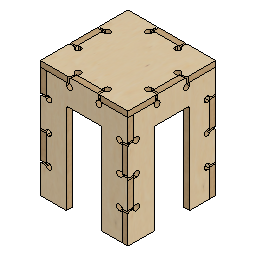
puzzleParam (Autodesk Fusion 360 design; units mm, degrees)
Autodesk Fusion 360 part; units mm, degrees
note: some values were not read from the file. Set by a fixed rule: which sketch regions a step uses.
sketch "Sketch1" plane through (0, 0, 0) normal (0, 0, 1) x (1, 0, 0)
  line L0 (-168.75, 168.75) -> (168.75, 168.75)
  line L1 (168.75, 168.75) -> (168.75, -168.75)
  line L2 (168.75, -168.75) -> (-168.75, -168.75)
  line L3 (-168.75, -168.75) -> (-168.75, 168.75)
  line L4 (-168.75, 168.75) -> (168.75, -168.75) construction
  line L5 (168.75, 168.75) -> (-168.75, -168.75) construction
  line L6 (146.75, -146.75) -> (-146.75, -146.75)
  line L7 (-146.75, -146.75) -> (-146.75, 146.75)
  line L8 (-146.75, 146.75) -> (146.75, 146.75)
  line L9 (146.75, 146.75) -> (146.75, -146.75)
  line L10 (-56.25, -168.75) -> (-56.25, 168.75)
  line L11 (56.25, -168.75) -> (56.25, 168.75)
  line L12 (168.75, -56.25) -> (-168.75, -56.25)
  line L13 (168.75, 56.25) -> (-168.75, 56.25)
  circle A0 centre (-56.25, -135.75) radius 11
  line L14 (-45.25, -135.75) -> (-45.25, -146.75)
  line L15 (0, 2.5) -> (0, 20)
  line L16 (45.25, -135.75) -> (45.25, -146.75)
  circle A1 centre (56.25, -135.75) radius 11
  circle A2 centre (135.75, -56.25) radius 11
  line L17 (135.75, -45.25) -> (146.75, -45.25)
  circle A3 centre (135.75, 56.25) radius 11
  line L18 (135.75, 45.25) -> (146.75, 45.25)
  circle A4 centre (56.25, 135.75) radius 11
  line L19 (45.25, 135.75) -> (45.25, 146.75)
  circle A5 centre (-56.25, 135.75) radius 11
  line L20 (-45.25, 135.75) -> (-45.25, 146.75)
  circle A6 centre (-135.75, 56.25) radius 11
  line L21 (-135.75, 45.25) -> (-146.75, 45.25)
  circle A7 centre (-135.75, -56.25) radius 11
  line L22 (-135.75, -45.25) -> (-146.75, -45.25)
  dimension "d7" = 337.5
  dimension "d8" = 337.5
  dimension "d9" = 22
  dimension "d12" = 112.5
  dimension "d13" = 0
  dimension "d16" = 0
  dimension "d17" = 112.5
  dimension "d18" = 22
  dimension "d20" = 360
  constraint horizontal L0
  constraint perpendicular L0 L1
  constraint parallel L0 L2
  constraint parallel L1 L3
  constraint coincident L4 origin
  constraint coincident L5 origin
  constraint coincident L10 A0.centre
  constraint tangent L6 A0
  constraint coincident A0 L14.start
  constraint coincident L6 L14.end
  constraint tangent A0 L14
  constraint perpendicular L6 L14
  constraint symmetric A0 L15 A1
  constraint symmetric L14.start L15 L16.start
  constraint symmetric L14.end L15 L16.end
  measures "d7" distance of L1.end L2.end
  measures "d8" distance of L0.end L1.end
  measures "d18" diameter of A0
extrude "Extrude1" add sketch "Sketch1" along normal blind 22 contours L0 L3 L7 L8 L10 L13 | L0 L1 L8 L9 L11 L13 | L7 L8 L10 L13 A5 A6 | L2 L3 L6 L7 L10 L12 | L8 L9 L11 L13 A3 A4 | L8 L10 L11 L13 A4 L19 A5 L20 | L6 L7 L10 L12 A0 A7 | L7 L10 L12 L13 A6 L21 A7 L22 | L10 L11 L12 L13 | L1 L2 L6 L9 L11 L12 | L9 L11 L12 L13 A2 L17 A3 L18 | L6 L10 L11 L12 A0 L14 L16 A1 | L6 L9 L11 L12 A1 A2 makes body 1
sketch "Sketch2" plane through (0, -168.75, 0) normal (0, -1, 0) x (1, 0, 0)
  line L0 (-168.75, 0) -> (-56.25, 0)
  line L1 (-56.25, 0) -> (-56.25, 22)
  line L2 (-56.25, 22) -> (-168.75, 22)
  line L3 (-168.75, 22) -> (-168.75, 0)
  line L4 (56.25, 0) -> (168.75, 0)
  line L5 (168.75, 0) -> (168.75, 22)
  line L6 (168.75, 22) -> (56.25, 22)
  line L7 (56.25, 22) -> (56.25, 0)
  line L8 (-168.75, 22) -> (168.75, 22)
  line L9 (168.75, 22) -> (168.75, -428)
  line L10 (168.75, -428) -> (-168.75, -428)
  line L11 (-168.75, -428) -> (-168.75, 22)
  line L12 (-56.25, -428) -> (-56.25, 22)
  line L13 (56.25, -428) -> (56.25, 22)
  line L14 (168.75, -315.5) -> (-168.75, -315.5)
  line L15 (168.75, -203) -> (-168.75, -203)
  line L16 (168.75, -90.5) -> (-168.75, -90.5)
  line L17 (-168.75, 0) -> (168.75, 0)
  line L18 (-146.75, -428) -> (-146.75, 22)
  line L19 (146.75, 22) -> (146.75, -428)
  circle A0 centre (-135.75, -315.5) radius 11
  circle A1 centre (-135.75, -203) radius 11
  circle A2 centre (-135.75, -90.5) radius 11
  line L20 (0, 1.75) -> (0, 22.5)
  circle A3 centre (135.75, -315.5) radius 11
  circle A4 centre (135.75, -203) radius 11
  circle A5 centre (135.75, -90.5) radius 11
  line L21 (-135.75, -304.5) -> (-146.75, -304.5)
  line L22 (-135.75, -214) -> (-146.75, -214)
  line L23 (-135.75, -79.5) -> (-146.75, -79.5)
  line L24 (135.75, -101.5) -> (146.75, -101.5)
  line L25 (135.75, -192) -> (146.75, -192)
  line L26 (135.75, -326.5) -> (146.75, -326.5)
  line L27 (-67.25, -428) -> (-67.25, -79.5)
  line L28 (67.25, -428) -> (67.25, -79.5)
  line L29 (67.25, -79.5) -> (-67.25, -79.5)
  circle A6 centre (-56.25, -11) radius 11
  line L30 (-67.25, -11) -> (-67.25, 0)
  circle A7 centre (56.25, -11) radius 11
  line L31 (67.25, -11) -> (67.25, 0)
  dimension "d24" = 337.5
  dimension "d25" = 450
  dimension "d28" = 112.5
  dimension "d29" = 0
  dimension "d32" = 0
  dimension "d33" = 112.5
  dimension "d36" = 22
  dimension "d39" = 0
  dimension "d40" = 112.5
  dimension "d44" = 22
  dimension "d57" = 11
  dimension "d58" = 11
  dimension "d59" = 11
  dimension "d60" = 22
  dimension "d61" = 22
  constraint horizontal L8
  constraint vertical L9
  constraint horizontal L10
  constraint vertical L11
  constraint coincident L2.end L3.start
  constraint coincident L0.start L3.end
  constraint coincident L4.end L5.start
  constraint coincident L14 A0.centre
  constraint tangent L18 A0
  constraint symmetric A0 L20 A3
  constraint symmetric A1 L20 A4
  constraint symmetric A2 L20 A5
  constraint coincident A0 L21.start
  constraint coincident L18 L21.end
  constraint tangent A0 L21
  constraint perpendicular L18 L21
  constraint coincident A1 L22.start
  constraint coincident L18 L22.end
  constraint tangent A1 L22
  constraint perpendicular L18 L22
  constraint coincident A2 L23.start
  constraint coincident L18 L23.end
  constraint tangent A2 L23
  constraint perpendicular L18 L23
  constraint coincident A5 L24.start
  constraint coincident L19 L24.end
  constraint tangent A5 L24
  constraint perpendicular L19 L24
  constraint coincident A4 L25.start
  constraint coincident L19 L25.end
  constraint tangent A4 L25
  constraint perpendicular L19 L25
  constraint coincident A3 L26.start
  constraint coincident L19 L26.end
  constraint tangent A3 L26
  constraint perpendicular L19 L26
  constraint coincident L12 A6.centre
  constraint tangent L17 A6
  constraint coincident A6 L30.start
  constraint coincident L17 L30.end
  constraint perpendicular L17 L30
  constraint tangent A6 L30
  constraint symmetric L20 A6 A7
  constraint symmetric L20 L30.start L31.start
  constraint symmetric L20 L30.end L31.end
  constraint perpendicular L27 L29
  constraint perpendicular L28 L29
  constraint coincident L10 L27.start
  constraint coincident L10 L28.start
  constraint coincident L10 L18.start
  constraint coincident L10 L19.end
  measures "d24" distance of L2.end L5.end
  measures "d25" distance of L2.end L10.end
  measures "d36" diameter of A0
  measures "d44" diameter of A6
  measures "d57" distance of L13 L28
  measures "d58" distance of L12 L27
  measures "d60" distance of L11 L18
  measures "d61" distance of L9 L19
extrude "Extrude2" add sketch "Sketch2" against normal blind 22 separate body contours L0 L12 L16 L17 L18 A2 L23 L27 L29 A6 L30 | L1 L7 L8 L12 L13 L17 | L12 L13 L17 L29 A6 A7 | L4 L13 L16 L17 L19 A5 L28 L29 A7 L31 | L11 L15 L16 L18 | L15 L16 L18 A1 A2 L27 | L4 L9 L16 L17 L19 | L10 L11 L14 L18 | L14 L15 L18 A0 A1 L21 L22 L27 | L15 L16 L19 A4 A5 L24 L25 L28 | L10 L14 L18 A0 L27 | L14 L15 L19 A3 A4 L28 | L9 L14 L15 L19 | L10 L14 L19 A3 L26 L28 makes body 2
move_face "OffsetFaces1" offset -0.0375 8 faces at (-56.25, -161.4167, 7.3333) (56.25, -161.4167, 14.6667) (-154.0833, 56.25, 7.3333) (-154.0833, -56.25, 7.3333) (56.25, 154.0833, 7.3333) (161.4167, -56.25, 7.3333) (-56.25, 154.0833, 7.3333) (161.4167, 56.25, 7.3333) on bodies 1
move_face "OffsetFaces2" offset -0.0375 8 faces at (-56.25, -154.0833, 7.3333) (56.25, -154.0833, 14.6667) (161.4167, -161.4167, -203) (161.4167, -161.4167, -90.5) (-154.0833, -154.0833, -90.5) (-154.0833, -154.0833, -315.5) (161.4167, -161.4167, -315.5) (-154.0833, -154.0833, -203) on bodies 2
fillet "Fillet1" radius 6.2857 8 edges at (-56.2875, -168.75, 11) (56.2875, -168.75, 11) (-168.75, 56.2875, 11) (-168.75, -56.2875, 11) (-56.2875, 168.75, 11) (56.2875, 168.75, 11) (168.75, 56.2875, 11) (168.75, -56.2875, 11) on bodies 1
fillet "Fillet1" radius 7.5429 8 edges at (146.7499, 56.2875, 11) (-56.2875, -146.7499, 11) (-146.7499, -56.2875, 11) (-146.7499, 56.2875, 11) (-56.2875, 146.7499, 11) (56.2875, 146.7499, 11) (146.7499, -56.2875, 11) (56.2875, -146.7499, 11) on bodies 1
fillet "Fillet1" radius 1.375 8 edges at (146.75, -45.25, 11) (146.75, 45.25, 11) (-45.25, 146.75, 11) (45.25, 146.75, 11) (45.25, -146.75, 11) (-45.25, -146.75, 11) (-146.75, -45.25, 11) (-146.75, 45.25, 11) on bodies 1
fillet "Fillet2" radius 7.5429 8 edges at (-56.2125, -157.75, -0.0001) (-146.7499, -157.75, -90.5375) (-146.7499, -157.75, -202.9625) (-146.7499, -157.75, -315.5375) (146.7499, -157.75, -315.4625) (146.7499, -157.75, -203.0375) (56.2125, -157.75, -0.0001) (146.7499, -157.75, -90.4625) on bodies 2
fillet "Fillet2" radius 6.2857 10 edges at (56.2125, -157.75, 22) (-56.2125, -157.75, 22) (-168.75, -157.75, -90.5375) (-168.75, -157.75, -202.9625) (-168.75, -157.75, -315.5375) (168.75, -157.75, -315.4625) (168.75, -157.75, -203.0375) (-67.25, -157.75, -79.5) (67.25, -157.75, -79.5) (168.75, -157.75, -90.4625) on bodies 2
fillet "Fillet2" radius 1.375 10 edges at (-67.25, -157.75, 0) (67.25, -157.75, 0) (146.75, -157.75, -192) (146.75, -157.75, -326.5) (67.25, -157.75, -428) (-67.25, -157.75, -428) (-146.75, -157.75, -304.5) (-146.75, -157.75, -214) (-146.75, -157.75, -79.5) (146.75, -157.75, -101.5) on bodies 2
pattern_circular "C-Pattern1" count 4 over 360 about axis through (0, 0, 1.75) along (0, 0, 1) of bodies 2 makes body 3 at (146.75, -123.7109, -394.106) makes body 4 at (123.7109, 168.75, -394.106) makes body 5 at (-146.75, 123.7109, -394.106)
copy_body "Body->Comp6" bodies 1 removing the originals makes body 6 in component "seat"
copy_body "Body->Comp7" bodies 2 removing the originals makes body 7 in component "leg1"
copy_body "Body->Comp8" bodies 3 removing the originals makes body 8 in component "leg2"
copy_body "Body->Comp9" bodies 4 removing the originals makes body 9 in component "leg3"
copy_body "Body->Comp10" bodies 5 removing the originals makes body 10 in component "leg4"
component "seat" placed x (1, 0, 0) y (0, 1, 0) z (0, 0, 1) at (0, 0, 0)
component "leg1" placed x (1, 0, 0) y (0, 1, 0) z (0, 0, 1) at (0, 0, 0)
component "leg2" placed x (1, 0, 0) y (0, 1, 0) z (0, 0, 1) at (0, 0, 0)
component "leg3" placed x (1, 0, 0) y (0, 1, 0) z (0, 0, 1) at (0, 0, 0)
component "leg4" placed x (1, 0, 0) y (0, 1, 0) z (0, 0, 1) at (0, 0, 0)
equation "vyska = 450 mm"
equation "sirka = vyska * 0.75"
equation "tloustka = 22 mm"
equation "prumer = tloustka * 1"
equation "zaobleniVstup = tloustka / 3.5"
equation "zaobleniHran = tloustka / 16"
equation "d7 = sirka"
equation "d8 = sirka"
equation "d9 = tloustka"
equation "d12 = sirka / 3"
equation "d17 = sirka / 3"
equation "d18 = prumer"
equation "d21 = tloustka"
equation "d24 = sirka"
equation "d25 = vyska"
equation "d28 = sirka / 3"
equation "d33 = sirka / 3"
equation "d36 = prumer"
equation "d40 = sirka / 3"
equation "d44 = prumer"
equation "d45 = -tloustka"
equation "d48 = zaobleniVstup"
equation "d50 = zaobleniVstup * 1.2"
equation "d52 = zaobleniVstup * 1.2"
equation "d54 = zaobleniVstup"
equation "d57 = tloustka / 2"
equation "d58 = tloustka / 2"
equation "d59 = tloustka / 2"
equation "d60 = tloustka"
equation "d61 = tloustka"
equation "d67 = zaobleniHran"
equation "d69 = zaobleniHran"
equation "d70 = -tolerance / 4"
equation "d71 = -tolerance / 4"
equation "tolerance = 0.15 mm"
named bodies: "seat", "leg1", "leg2", "leg3", "leg4"
